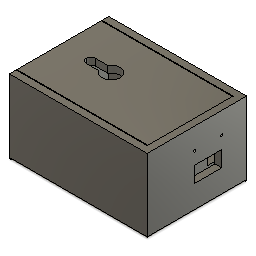
Ledstrip-controller-case (Autodesk Fusion 360 design; units mm, degrees)
Autodesk Fusion 360 part; units mm, degrees
note: some values were not read from the file. Set by a fixed rule: which sketch regions a step uses.
sketch "Sketch1" plane through (0, 0, 0) normal (0, 1, 0) x (1, 0, 0) in component "Logic board"
  line L0 (0, 0) -> (46, 0)
  line L1 (46, 0) -> (46, -38)
  line L2 (46, -38) -> (0, -38)
  line L3 (0, -38) -> (0, 0)
  line L4 (46, 0) -> (44.5, 0)
  line L5 (44.5, 0) -> (44.5, -4)
  line L6 (44.5, -4) -> (46, -4)
  line L7 (46, -4) -> (46, 0)
  line L8 (44.5, -4) -> (-7.5, -4)
  line L9 (-7.5, -4) -> (-7.5, -24.5)
  line L10 (-7.5, -24.5) -> (44.5, -24.5)
  line L11 (44.5, -24.5) -> (44.5, -4)
  line L12 (46, -38) -> (26, -38)
  line L13 (26, -38) -> (26, -29)
  line L14 (26, -29) -> (46, -29)
  line L15 (46, -29) -> (46, -38)
  line L16 (44.5, -9.9563) -> (38, -9.9563)
  line L17 (38, -9.9563) -> (38, -17.9563)
  line L18 (38, -17.9563) -> (44.5, -17.9563)
  line L19 (44.5, -17.9563) -> (44.5, -9.9563)
  dimension "d1" = 46
  dimension "d2" = 38
  dimension "d3" = 1.5
  dimension "d4" = 4
  dimension "d5" = 52
  dimension "d6" = 20.5
  dimension "d7" = 20
  dimension "d8" = 9
  dimension "d13" = 8
  constraint horizontal L0
  constraint vertical L1
  constraint horizontal L2
  constraint vertical L3
  constraint coincident L0.start L3.end
  constraint horizontal L4
  constraint vertical L5
  constraint horizontal L6
  constraint vertical L7
  constraint horizontal L8
  constraint vertical L9
  constraint horizontal L10
  constraint vertical L11
  constraint horizontal L12
  constraint vertical L13
  constraint horizontal L14
  constraint vertical L15
  constraint horizontal L16
  constraint vertical L17
  constraint horizontal L18
  constraint vertical L19
  constraint coincident L11 L16.start
  measures "d1" distance of L0.start L0.end
  measures "d2" distance of L0.start L2.end
  measures "d3" distance of L0.end L4.end
  measures "d4" distance of L0.end L6.end
  measures "d5" distance of L5.end L8.end
  measures "d6" distance of L5.end L10.end
  measures "d7" distance of L1.end L12.end
  measures "d8" distance of L1.end L14.end
  measures "d13" distance of L16.start L18.end
extrude "Extrude3" add sketch "Sketch1" along normal blind 11 contours L11 L16 L17 L18 L19 makes body 1 in component "Logic board"
extrude "Extrude1" add sketch "Sketch1" along normal blind 4 separate body contours L0 L3 L5 L8 | L0 L1 L4 L5 L6 L7 | L3 L8 L10 L11 L16 L17 L18 | L1 L2 L3 L6 L10 L11 L13 L14 L19 | L11 L16 L17 L18 L19 | L1 L2 L12 L13 L14 L15 makes body 2 in component "Logic board"
extrude "Extrude2" add sketch "Sketch1" along normal blind 7.5 separate body contours L3 L8 L10 L11 L16 L17 L18 | L3 L8 L9 L10 | L11 L16 L17 L18 L19 makes body 3 in component "Logic board"
extrude "Extrude4" add sketch "Sketch1" along normal blind 25 separate body contours L1 L2 L12 L13 L14 L15 makes body 4 in component "Logic board"
combine "Combine1" operation add target body 1 tool bodies 3 4 2 in component "Logic board"
sketch "Floorplan" plane through (0, 0, 0) normal (0, 1, 0) x (1, 0, 0) in component "Old Housing"
  line L0 (45, 2) -> (48, 2)
  line L1 (48, 2) -> (48, -42)
  line L2 (48, -42) -> (45, -42)
  line L3 (45, -40) -> (45, -2)
  line L4 (48, 2) -> (-10, 2)
  line L5 (-10, 2) -> (-10, -2)
  line L6 (-8, -2) -> (45, -2)
  line L7 (48, -2) -> (48, 2)
  line L8 (-10, 2) -> (48, 2)
  line L9 (48, 2) -> (48, -42)
  line L10 (48, -42) -> (-10, -42)
  line L11 (-10, -42) -> (-10, 2)
  line L12 (46, 0) -> (46, -40)
  line L13 (46, -40) -> (-8, -40)
  line L14 (-8, -40) -> (-8, 0)
  line L15 (46, 0) -> (-8, 0)
  line L16 (10, -27) -> (-8, -27)
  line L17 (-8, -27) -> (-8, -40)
  line L18 (-8, -40) -> (10, -40)
  line L19 (10, -40) -> (10, -27)
  line L20 (-1, -39) -> (-4, -39)
  line L21 (-4, -39) -> (-4, -28)
  line L22 (-4, -28) -> (-1, -28)
  line L23 (-1, -28) -> (-1, -39)
  dimension "d18" = 44
  dimension "d19" = 2
  dimension "d20" = 18
  constraint horizontal L0
  constraint vertical L1
  constraint horizontal L2
  constraint vertical L3
  constraint horizontal L4
  constraint vertical L5
  constraint horizontal L6
  constraint vertical L7
  constraint horizontal L8
  constraint vertical L9
  constraint horizontal L10
  constraint vertical L11
  constraint coincident L13 L3.start
  constraint coincident L14 L6.start
  constraint horizontal L16
  constraint vertical L17
  constraint horizontal L18
  constraint vertical L19
  constraint horizontal L20
  constraint vertical L21
  constraint horizontal L22
  constraint vertical L23
  measures "d18" distance of L0.start L2.end
  measures "d20" distance of L16.start L16.end
sketch "floorplan" plane through (0, 0, 0) normal (0, 1, 0) x (1, 0, 0) in component "Housing"
  line L0 (46, 0) -> (-12, 0)
  line L1 (-12, 0) -> (-12, -38)
  line L2 (-12, -38) -> (46, -38)
  line L3 (46, -38) -> (46, 0)
  line L4 (49, 3) -> (-15, 3)
  line L5 (-15, 3) -> (-15, -41)
  line L6 (-15, -41) -> (49, -41)
  line L7 (49, -41) -> (49, 3)
  line L8 (-4, -27) -> (10, -27)
  line L9 (10, -27) -> (10, -38)
  line L10 (10, -38) -> (-4, -38)
  line L11 (-4, -38) -> (-4, -27)
  line L12 (-4, -27) -> (-1, -27)
  line L13 (-1, -27) -> (-1, -38)
  line L14 (-1, -38) -> (-4, -38)
  line L15 (-4, -38) -> (-4, -27)
  line L16 (-4, -2) -> (46, -2)
  line L17 (46, -2) -> (46, 0)
  line L18 (46, 0) -> (-4, 0)
  line L19 (-4, 0) -> (-4, -2)
  line L20 (46, -18) -> (-4, -18)
  line L21 (-4, -18) -> (-4, -10)
  line L22 (-4, -10) -> (46, -10)
  line L23 (46, -10) -> (46, -18)
  line L24 (-4, -10) -> (-1, -10)
  line L25 (-1, -10) -> (-1, -18)
  line L26 (-1, -18) -> (-4, -18)
  line L27 (-4, -18) -> (-4, -10)
  line L28 (-4, 0) -> (-1, 0)
  line L29 (-1, 0) -> (-1, -2)
  line L30 (-1, -2) -> (-4, -2)
  line L31 (-4, -2) -> (-4, 0)
  line L32 (-12, 0) -> (-12, 3)
  line L33 (-12, -38) -> (-12, -41)
  line L34 (46, 0) -> (45, 0)
  line L35 (45, 0) -> (45, -38)
  line L36 (45, -38) -> (46, -38)
  line L37 (46, -38) -> (46, 0)
  dimension "d65" = 3
  constraint horizontal L0
  constraint vertical L1
  constraint horizontal L2
  constraint vertical L3
  constraint horizontal L8
  constraint vertical L9
  constraint horizontal L10
  constraint vertical L11
  constraint coincident L2 L9.end
  constraint horizontal L12
  constraint vertical L13
  constraint horizontal L14
  constraint vertical L15
  constraint coincident L2 L13.end
  constraint horizontal L16
  constraint vertical L17
  constraint horizontal L18
  constraint vertical L19
  constraint horizontal L20
  constraint vertical L21
  constraint horizontal L22
  constraint vertical L23
  constraint coincident L3 L20.start
  constraint horizontal L24
  constraint vertical L25
  constraint horizontal L26
  constraint vertical L27
  constraint coincident L20 L25.end
  constraint horizontal L28
  constraint vertical L29
  constraint horizontal L30
  constraint vertical L31
  constraint coincident L16 L29.end
  constraint coincident L4 L32.end
  constraint perpendicular L4 L32
  constraint coincident L6 L33.end
  constraint perpendicular L6 L33
  constraint horizontal L34
  constraint vertical L35
  constraint horizontal L36
  constraint vertical L37
  constraint coincident L2 L35.end
extrude "Extrude1'" add sketch "Floorplan" against normal blind 2 separate body contours L0 L1 L2 L4 L5 L7 L8 L9 L10 L11 | L3 L6 L13 L14 L16 L19 | L3 L6 L12 L13 L14 L15 | L13 L14 L16 L17 L18 L19 | L20 L21 L22 L23 makes body 5 in component "Old Housing"
extrude "Extrude2'" add sketch "Floorplan" along normal blind 3.5 separate body contours L0 L1 L2 L4 L5 L7 L8 L9 L10 L11 | L3 L6 L12 L13 L14 L15 | L13 L14 L16 L17 L18 L19 | L20 L21 L22 L23 makes body 6 in component "Old Housing"
extrude "Extrude3'" add sketch "Floorplan" along normal blind 28 separate body contours L0 L1 L2 L4 L5 L7 L8 L9 L10 L11 makes body 7 in component "Old Housing"
combine "Combine1'" operation add target body 5 tool bodies 7 6 in component "Old Housing"
sketch "usb entree" plane through (46, 0, 0) normal (-1, 0, 0) x (0, 0, 1) in component "Old Housing"
  line L0 (0, 3.5) -> (40, 3.5)
  line L1 (40, 3.5) -> (40, 28)
  line L2 (40, 28) -> (0, 28)
  line L3 (0, 28) -> (0, 3.5)
  line L4 (10, 13.2) -> (17.964, 13.2)
  line L5 (17.964, 13.2) -> (17.964, 9.6949)
  line L6 (17.964, 9.6949) -> (10, 9.6949)
  line L7 (10, 9.6949) -> (10, 13.2)
  line L8 (19.964, 7.6949) -> (8, 7.6949)
  line L9 (8, 7.6949) -> (8, 15.2)
  line L10 (8, 15.2) -> (19.964, 15.2)
  line L11 (19.964, 15.2) -> (19.964, 7.6949)
  dimension "d27" = -2
  constraint horizontal L4
  constraint vertical L5
  constraint horizontal L6
  constraint vertical L7
extrude "Extrude4'" cut sketch "usb entree" along normal mid plane 6 contours L4 L5 L6 L7 | L8 L9 L10 L11 bodies 5 in component "Old Housing"
sketch "Sketch1 (2)" plane through (0, 0, -2) normal (0, 0, -1) x (-1, 0, 0) in component "Old Buttons"
  line L0 (10, -2) -> (10, 28)
  line L1 (10, 28) -> (-48, 28)
  line L2 (-48, 28) -> (-48, -2)
  line L3 (-48, -2) -> (10, -2)
  circle A0 centre (-25, 18.5) radius 5
  circle A1 centre (-13, 18.5) radius 5
  circle A2 centre (-25, 18.5) radius 0.5
  circle A3 centre (-13, 18.5) radius 0.5
  dimension "d30" = 10
  dimension "d31" = 10
  dimension "d32" = 1
  dimension "d33" = 1
  constraint concentric A0 A2
  constraint concentric A1 A3
  measures "d30" diameter of A0
  measures "d31" diameter of A1
  measures "d32" diameter of A2
  measures "d33" diameter of A3
extrude "Extrude1''" add sketch "Sketch1 (2)" against normal blind 15 separate body contours A2 | A3 makes body 8 at (25.4391, 18.7391, 8) makes body 9 at (13.4607, 18.3058, 8) in component "Old Buttons"
extrude "Extrude2''" add sketch "Sketch1 (2)" along normal blind 4 contours A0 | A1 | A2 | A3 bodies 8 9 in component "Old Buttons"
fillet "Fillet1" radius 4 2 edges at (29.6616, 16.6919, -6) (17.6616, 16.6919, -6) on bodies 8 9 in component "Old Buttons"
combine "Combine2" operation cut target body 5 tool bodies 8 9 keep tools in component "Old Housing"
sketch "Sketch3" plane through (-8, 0, 0) normal (1, 0, 0) x (0, 0, -1) in component "Old Housing"
  line L0 (-2, 3.5) -> (0, 3.5)
  line L1 (0, 3.5) -> (0, 28)
  line L2 (0, 28) -> (-40, 28)
  line L3 (-40, 28) -> (-40, 3.5)
  line L4 (-40, 3.5) -> (-27, 3.5)
  line L5 (-27, 3.5) -> (-27, 0)
  line L6 (-27, 0) -> (-2, 0)
  line L7 (-2, 0) -> (-2, 3.5)
  line L8 (0, 28) -> (-40, 28)
  line L9 (-40, 28) -> (-40, 0)
  line L10 (-40, 0) -> (0, 0)
  line L11 (0, 0) -> (0, 28)
  dimension "d39" = 28
  constraint horizontal L8
  constraint vertical L9
  constraint horizontal L10
  constraint vertical L11
  constraint coincident L1.end L2.start
  measures "d39" distance of L1.end L10.end
extrude "Extrude5" cut sketch "Sketch3" along normal mid plane 8 bodies 5 in component "Old Housing"
sketch "Sketch1 (3)" plane through (0, 28, 0) normal (0, 1, 0) x (-1, 0, 0) in component "Old Lid"
  line L0 (-46, 40) -> (10, 40)
  line L1 (10, 40) -> (10, 42)
  line L2 (10, 42) -> (-48, 42)
  line L3 (-48, 42) -> (-48, -2)
  line L4 (-48, -2) -> (10, -2)
  line L5 (10, -2) -> (10, 0)
  line L6 (10, 0) -> (-46, 0)
  line L7 (-46, 0) -> (-46, 40)
  line L8 (-46, 0) -> (10, 0)
  line L9 (10, 0) -> (10, 40)
  line L10 (10, 40) -> (-46, 40)
  line L11 (-46, 40) -> (-46, 0)
  line L12 (10, 0) -> (8, 0)
  line L13 (8, 0) -> (8, 40)
  line L14 (8, 40) -> (10, 40)
  line L15 (10, 40) -> (10, 0)
  constraint horizontal L8
  constraint vertical L9
  constraint horizontal L10
  constraint vertical L11
  constraint coincident L0.end L1.start
  constraint coincident L6.end L7.start
  constraint horizontal L12
  constraint vertical L13
  constraint horizontal L14
  constraint vertical L15
  constraint coincident L0 L13.end
  constraint coincident L5.end L6.start
extrude "Extrude1'''" add sketch "Sketch1 (3)" against normal blind 2 separate body contours L0 L6 L7 L8 L10 L11 L13 | L0 L6 L8 L9 L10 L12 L13 L14 L15 makes body 10 in component "Old Lid"
extrude "Extrude2'''" add sketch "Sketch1 (3)" against normal blind 27.5 separate body contours L0 L6 L8 L9 L10 L12 L13 L14 L15 makes body 11 in component "Old Lid"
combine "Combine1''" operation add target body 10 tool bodies 11 keep tools in component "Old Lid"
combine "Combine2'" operation add target body 10 tool bodies 11 in component "Old Lid"
sketch "Sketch2" plane through (-10, 0, 0) normal (-1, 0, 0) x (0, 0, 1) in component "Old Lid"
  line L0 (40, 28) -> (0, 28)
  line L1 (0, 28) -> (0, 0.5)
  line L2 (0, 0.5) -> (40, 0.5)
  line L3 (40, 0.5) -> (40, 28)
  circle A0 centre (0, 27.1414) radius 0.5
  circle A1 centre (40, 26.9619) radius 0.5
  dimension "d48" = 1
  dimension "d49" = 1
  constraint coincident L1 A0.centre
  constraint coincident L3 A1.centre
  measures "d48" diameter of A0
  measures "d49" diameter of A1
extrude "Extrude3''" add sketch "Sketch2" against normal blind 56 separate body contours L3 A1 | L3 A1 | L1 A0 | L1 A0 makes body 12 at (8.6667, 27.4618, 39.991) makes body 13 at (27.3333, 26.999, 0.4793) in component "Old Lid"
copy_body "CopyPasteBodies3" bodies 12 makes body 14 in component "Old Lid"
move_body "Move3" bodies 14 to x (1, 0, 0) y (0, 1, 0) z (0, 0, 1) at (0, 0, 0) in component "Old Lid"
copy_body "CopyPasteBodies4" bodies 13 makes body 15 in component "Old Lid"
move_body "Move4" bodies 15 to x (1, 0, 0) y (0, 1, 0) z (0, 0, 1) at (0, 0, 0.5) in component "Old Lid"
move_body "Move5" bodies 14 to x (1, 0, 0) y (0, 1, 0) z (0, 0, 1) at (0, 0, 0.5) in component "Old Lid"
move_body "Move6" bodies 15 to x (1, 0, 0) y (0, 1, 0) z (0, 0, 1) at (0, 0, -0.5) in component "Old Lid"
move_body "Move7" bodies 14 to x (1, 0, 0) y (0, 1, 0) z (0, 0, 1) at (0, 0, -0.5) in component "Old Lid"
combine "Combine5" operation add target body 10 tool bodies 14 15 in component "Old Lid"
combine "Combine3" operation cut target body 5 tool bodies 12 13 in component "Old Housing"
sketch "Sketch3 (2)" plane through (-8, 0, 0) normal (1, 0, 0) x (0, 0, -1) in component "Old Lid"
  line L0 (0, 26) -> (-40, 26)
  line L1 (-40, 26) -> (-40, 0.5)
  line L2 (-40, 0.5) -> (0, 0.5)
  line L3 (0, 0.5) -> (0, 26)
  line L4 (-27.0736, 0.5) -> (-37, 0.5)
  line L5 (-37, 0.5) -> (-37, 7)
  line L6 (-37, 7) -> (-27.0736, 7)
  line L7 (-27.0736, 7) -> (-27.0736, 0.5)
  constraint horizontal L4
  constraint vertical L5
  constraint horizontal L6
  constraint vertical L7
  constraint coincident L2 L4.start
extrude "Extrude4''" cut sketch "Sketch3 (2)" along normal mid plane 6 contours L2 L4 L5 L6 L7 bodies 10 in component "Old Lid"
fillet "Fillet1'" radius 1 1 edges at (-9, 7, 27.0736) on bodies 10 in component "Old Lid"
fillet "Fillet2" radius 1 1 edges at (-9, 7, 37) on bodies 10 in component "Old Lid"
extrude "Extrude6" add sketch "Floorplan" along normal blind 4.5 contours L20 L21 L22 L23 bodies 5 in component "Old Housing"
copy_body "CopyPasteBodies1" bodies 9 makes body 16
move_body "Move1" bodies 16 to x (0, 0, 1) y (0, 1, 0) z (-1, 0, 0) at (46, 2, -5)
copy_body "CutPasteBodies1" bodies 16 removing the originals makes body 17 in component "Old Buttons"
copy_body "CopyPasteBodies2" bodies 8 makes body 18
move_body "Move2" bodies 18 to x (0, 0, 1) y (0, 1, 0) z (-1, 0, 0) at (46, 2, -5)
copy_body "CutPasteBodies2" bodies 18 removing the originals makes body 19 in component "Old Buttons"
combine "Combine4" operation cut target body 5 tool bodies 17 19 keep tools in component "Old Housing"
fillet "Fillet3" radius 1 1 edges at (-8, 26, 20) on bodies 10 in component "Old Lid"
fillet "Fillet2'" radius 1 3 edges at (19, 28, -2) (48, 28, 20) (19, 28, 42) on bodies 5 in component "Old Housing"
fillet "Fillet3'" radius 1 9 edges at (-7, 0, 40) (27.5, 0, 40) (-4, 0, 33.5) (3, 0, 27) (45, 0, 21) (20.5, 0, 2) (-4, 0, 1) (-7, 0, 0) (10, 0, 33.5) on bodies 5 in component "Old Housing"
fillet "Fillet5" radius 1 2 edges at (-9, 0.5, 40) (-9, 0.5, 0) on bodies 10 in component "Old Lid"
extrude "Extrude1''''" add sketch "floorplan" against normal blind 3 separate body contours L0 L3 L16 L17 L18 L34 L35 L37 | L0 L2 L3 L4 L6 L7 L10 L14 L17 L18 L23 L28 L32 L33 L34 L36 L37 | L0 L16 L18 L29 L35 | L3 L16 L22 L35 L37 | L0 L16 L18 L19 L28 L29 L30 L31 | L0 L1 L2 L8 L9 L11 L12 L15 L16 L19 L20 L21 L22 L24 L26 L27 L30 L31 L35 | L3 L20 L22 L23 L35 L37 | L20 L22 L25 L35 | L2 L3 L20 L35 L36 L37 | L20 L21 L22 L24 L25 L26 L27 | L2 L8 L10 L11 L12 L13 L14 L15 | L2 L8 L9 L10 L13 makes body 20 in component "Housing"
extrude "Extrude2''''" add sketch "floorplan" along normal blind 30 contours L0 L2 L3 L4 L6 L7 L10 L14 L17 L18 L23 L28 L32 L33 L34 L36 L37 bodies 20 in component "Housing"
extrude "Extrude3'''" add sketch "floorplan" along normal blind 3 separate body contours L0 L3 L16 L17 L18 L34 L35 L37 | L0 L16 L18 L29 L35 | L3 L16 L22 L35 L37 | L3 L20 L22 L23 L35 L37 | L20 L22 L25 L35 | L2 L3 L20 L35 L36 L37 | L2 L8 L9 L10 L13 makes body 21 at (6.3333, 0, 34.3333) makes body 22 at (14.3333, 0, 12.6667) in component "Housing"
extrude "Extrude4'''" add sketch "floorplan" along normal blind 4 separate body contours L0 L16 L18 L19 L28 L29 L30 L31 | L20 L21 L22 L24 L25 L26 L27 | L2 L8 L10 L11 L12 L13 L14 L15 makes body 23 at (-3, 1.3333, 2) makes body 24 at (-1, 1.3333, 12.6667) makes body 25 at (-4, 1.3333, 34.3333) in component "Housing"
extrude "Extrude5'" add sketch "floorplan" along normal blind 1 separate body contours L0 L3 L16 L17 L18 L34 L35 L37 | L3 L16 L22 L35 L37 | L3 L20 L22 L23 L35 L37 | L2 L3 L20 L35 L36 L37 makes body 26 in component "Housing"
move_body "Move1'" bodies 26 to x (1, 0, 0) y (0, 1, 0) z (0, 0, 1) at (0, 5, 0) in component "Housing"
combine "Combine1'''" operation add target body 20 tool bodies 25 24 22 26 21 23 in component "Housing"
sketch "Sketch1 (4)" plane through (0, 0, 0) normal (0, 1, 0) x (1, 0, 0) in component "Lid"
  line L0 (46, 0) -> (-12, 0)
  line L1 (-12, 0) -> (-12, -38)
  line L2 (-12, -38) -> (46, -38)
  line L3 (46, -38) -> (46, 0)
  line L4 (-12, 0) -> (-9, 0)
  line L5 (-9, 0) -> (-9, -38)
  line L6 (-9, -38) -> (-12, -38)
  line L7 (-12, -38) -> (-12, 0)
  line L8 (-9, -38) -> (-12, -38)
  line L9 (-12, -38) -> (-12, -32)
  line L10 (-12, -32) -> (-9, -32)
  line L11 (-9, -32) -> (-9, -38)
  circle A0 centre (10, -18) radius 4
  line L12 (10, -16) -> (1, -16)
  line L13 (-1, -18) -> (-1, -18.0001)
  line L14 (1, -20) -> (10, -20)
  line L15 (10, -20) -> (10, -16)
  arc A1 (1, -16) -> (-1, -18) centre (1, -18) ccw
  arc A2 (-1, -18.0001) -> (1, -20) centre (1, -18) ccw
  point P0 (-1, -16)
  dimension "d76" = 6
  dimension "d83" = 8
  dimension "d84" = 11
  dimension "d85" = 4
  dimension "d86" = 2
  constraint horizontal L0
  constraint vertical L1
  constraint horizontal L2
  constraint vertical L3
  constraint horizontal L4
  constraint vertical L5
  constraint horizontal L6
  constraint vertical L7
  constraint coincident L2 L5.end
  constraint horizontal L8
  constraint vertical L9
  constraint horizontal L10
  constraint vertical L11
  constraint horizontal L12
  constraint horizontal L14
  constraint vertical L15
  constraint coincident P0 L12
  constraint tangent L12 A1
  constraint tangent L14 A2
  constraint equal A1 A2
  measures "d76" distance of L5.end L10.end
  measures "d83" diameter of A0
  measures "d84" distance of L12.start P0
  measures "d85" distance of L12.start L14.end
  measures "d86" radius of A1
extrude "Extrude4''''" add sketch "Sketch1 (4)" along normal mid plane 8 separate body contours A0 L12 L14 L15 | A0 L12 L14 L15 | A0 L12 L14 A1 A2 makes body 27 in component "Lid"
extrude "Extrude1'''''" add sketch "Sketch1 (4)" along normal blind 3 separate body contours L0 L2 L3 L5 L11 | L0 L1 L4 L5 L7 L10 | L1 L2 L5 L6 L7 L8 L9 L10 L11 | A0 L12 L14 L15 | A0 L12 L14 L15 | A0 L12 L14 A1 A2 makes body 28 in component "Lid"
extrude "Extrude2'''''" add sketch "Sketch1 (4)" against normal blind 26.5 contours L0 L1 L4 L5 L7 L10 bodies 28 in component "Lid"
extrude "Extrude3''''" add sketch "Sketch1 (4)" against normal blind 20.5 contours L1 L2 L5 L6 L7 L8 L9 L10 L11 bodies 28 in component "Lid"
move_body "Move1''" bodies 28 to x (1, 0, 0) y (0, 1, 0) z (0, 0, 1) at (0, 27, 0) in component "Lid"
move_body "Move2'" bodies 27 to x (1, 0, 0) y (0, 1, 0) z (0, 0, 1) at (0, 29, 0) in component "Lid"
combine "Combine1''''" operation cut target body 28 tool bodies 27 in component "Lid"
sketch "Sketch2 (2)" plane through (-12, 0, 0) normal (-1, 0, 0) x (0, 0, 1) in component "Lid"
  line L0 (38, 6.5) -> (38, 30)
  line L1 (38, 30) -> (0, 30)
  line L2 (0, 30) -> (0, 0.5)
  line L3 (0, 0.5) -> (32, 0.5)
  line L4 (32, 0.5) -> (32, 6.5)
  line L5 (32, 6.5) -> (38, 6.5)
  circle A0 centre (0, 28.5) radius 1
  circle A1 centre (38, 28.5) radius 1
  constraint coincident L0 A1.centre
extrude "Extrude5''" add sketch "Sketch2 (2)" against normal blind 55 separate body contours L0 A1 | L0 A1 | L2 A0 | L2 A0 makes body 29 at (6.3333, 28.5996, 0.995) makes body 30 at (6.3333, 29.4115, 37.5887) in component "Lid"
move_body "Move3'" bodies 29 30 to x (1, 0, 0) y (0, 1, 0) z (0, 0, 1) at (2, 0, 0) in component "Lid"
combine "Combine2''" operation cut target body 20 tool bodies 29 30 keep tools in component "Housing"
move_face "OffsetFaces1" offset -0.3 1 faces at (8.3333, 29, 38) on bodies 28 in component "Lid"
move_face "OffsetFaces2" offset -0.3 1 faces at (8.3333, 29, 0) on bodies 28 in component "Lid"
move_body "Move4'" bodies 29 to x (1, 0, 0) y (0, 1, 0) z (0, 0, 1) at (0, 0, 0.3) in component "Lid"
move_body "Move5'" bodies 30 to x (1, 0, 0) y (0, 1, 0) z (0, 0, 1) at (0, 0, -0.3) in component "Lid"
combine "Combine2'''" operation add target body 28 tool bodies 29 30 in component "Lid"
fillet "Fillet1''" radius 1 1 edges at (45, 28.5, 38.7) on bodies 28 in component "Lid"
fillet "Fillet2''" radius 1 1 edges at (45, 28.5, -0.7) on bodies 28 in component "Lid"
fillet "Fillet3''" radius 1 1 edges at (-10, 28.5, -0.7) on bodies 28 in component "Lid"
fillet "Fillet4" radius 1 1 edges at (-10, 28.5, 38.7) on bodies 28 in component "Lid"
sketch "Sketch2 (3)" plane through (46, 0, 0) normal (-1, 0, 0) x (0, 0, -1) in component "Housing"
  line L0 (-20, -15) -> (-8, -15)
  line L1 (-8, -15) -> (-8, -8)
  line L2 (-8, -8) -> (-20, -8)
  line L3 (-20, -8) -> (-20, -15)
  circle A0 centre (-20, -20.5) radius 0.5
  circle A1 centre (-8, -20.5) radius 0.5
  constraint horizontal L0
  constraint vertical L1
  constraint horizontal L2
  constraint vertical L3
sketch "Sketch3 (3)" plane through (0, 0, -3) normal (0, 0, -1) x (-1, 0, 0) in component "Housing"
  line L0 (-49, 30) -> (-49, -3)
  line L1 (-49, -3) -> (12, -3)
  line L2 (12, -3) -> (12, 30)
  line L3 (12, 30) -> (-49, 30)
  circle A0 centre (-25, 18.5) radius 0.5
  circle A1 centre (-13, 18.5) radius 0.5
extrude "Extrude6'" cut sketch "Sketch3 (3)" against normal blind 3 contours A0 | A1 bodies 20 in component "Housing"
extrude "Extrude7" cut sketch "Sketch2 (3)" against normal blind 3 bodies 20 in component "Housing"
fillet "Fillet1'''" radius 1 3 edges at (-4, 4, 1) (-4, 4, 14) (-4, 4, 32.5) on bodies 20 in component "Housing"
fillet "Fillet2'''" radius 1 4 edges at (18.5, -3, 41) (-12, -3, 19) (18.5, -3, -3) (49, -3, 19) on bodies 20 in component "Housing"
component "Housing" placed x (1, 0, 0) y (0, 1, 0) z (0, 0, 1) at (0, 0, 0)
component "Logic board" placed x (1, 0, 0) y (0, 1, 0) z (0, 0, 1) at (0, 0, 0)
component "Lid" placed x (1, 0, 0) y (0, 1, 0) z (0, 0, 1) at (0, 0, 0)
component "Old Buttons" placed x (1, 0, 0) y (0, 1, 0) z (0, 0, 1) at (0, 0, 0)
component "Old Housing" placed x (1, 0, 0) y (0, 1, 0) z (0, 0, 1) at (0, 0, 0)
component "Old Lid" placed x (1, 0, 0) y (0, 1, 0) z (0, 0, 1) at (0, 0, 0)
named bodies: "Logic Board", "Housing", "ButtonLeft", "ButtonRight", "Lid", "ButtonRightFront", "ButtonLeftFront", "New Housing", "New Lid"
